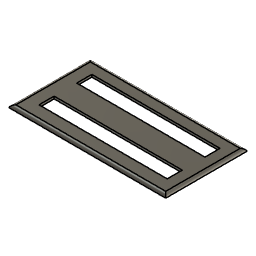
Battery Tray Plate (Autodesk Fusion 360 design; units mm, degrees)
Autodesk Fusion 360 part; units mm, degrees
box "BoxPrimitive1" add length 108 width 208 height 3.2 placed x (0, 1, 0) y (-1, 0, 0) z (0, 0, 1) at (208, 0, 0)
fillet "Fillet1" radius 5 4 edges at (0, 54, 3.2) (104, 108, 3.2) (208, 54, 3.2) (104, 0, 3.2)
sketch "Sketch8" plane through (0, 0, 3.2) normal (0, 0, 1) x (-1, 0, 0)
  line L0 (-203.3352, -103.3352) -> (-4.6648, -103.3352)
  line L1 (-4.6648, -103.3352) -> (-4.6648, -4.6648)
  line L2 (-4.6648, -4.6648) -> (-203.3352, -4.6648)
  line L3 (-203.3352, -4.6648) -> (-203.3352, -103.3352)
  line L4 (-20, -90) -> (-190, -90)
  line L5 (-190, -90) -> (-190, -70)
  line L6 (-190, -70) -> (-20, -70)
  line L7 (-20, -70) -> (-20, -90)
  line L8 (-20, -40) -> (-190, -40)
  line L9 (-190, -40) -> (-190, -20)
  line L10 (-190, -20) -> (-20, -20)
  line L11 (-20, -20) -> (-20, -40)
  constraint horizontal L4
  constraint vertical L5
  constraint horizontal L6
  constraint vertical L7
  constraint horizontal L8
  constraint vertical L9
  constraint horizontal L10
  constraint vertical L11
extrude "Extrude1" cut sketch "Sketch8" against normal blind 10 contours L4 L5 L6 L7 | L8 L9 L10 L11
